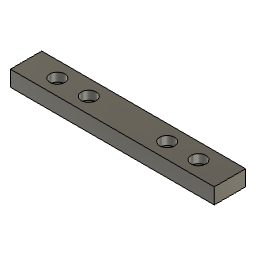
연습예제_1 (Autodesk Fusion 360 design; units mm, degrees)
Autodesk Fusion 360 part; units mm, degrees
sketch "Sketch1" plane through (0, 0, 0) normal (0, 0, 1) x (1, 0, 0)
  line L0 (-65, 20) -> (65, 20)
  line L1 (65, 20) -> (65, 0)
  line L2 (65, 0) -> (-65, 0)
  line L3 (-65, 0) -> (-65, 20)
  dimension "d1" = 130
  dimension "d2" = 20
  constraint horizontal L0
  constraint vertical L1
  constraint horizontal L2
  constraint vertical L3
  constraint midpoint origin L2
  measures "d1" distance of L0.start L0.end
  measures "d2" distance of L0.end L1.end
extrude "Extrude1" add sketch "Sketch1" along normal blind 10
sketch "Sketch3" plane through (0, 0, 10) normal (0, 0, 1) x (-1, 0, 0)
  line L0 (65, -20) -> (65, 0)
  line L1 (65, -10) -> (45, -10)
  line L2 (45, -10) -> (25, -10)
  line L3 (-65, 0) -> (-65, -20)
  line L4 (-65, -10) -> (-45, -10)
  line L5 (-45, -10) -> (-25, -10)
  point P0 (65, -20)
  dimension "d10" = 20
  dimension "d11" = 20
  dimension "d12" = 20
  dimension "d13" = 20
  constraint midpoint L0 L1.start
  constraint perpendicular L0 L1
  constraint parallel L1 L2
  constraint midpoint L3 L4.start
  constraint perpendicular L3 L4
  constraint parallel L4 L5
  measures "d10" distance of L1.start L1.end
  measures "d11" distance of L1.end L2.end
  measures "d12" distance of L4.start L4.end
  measures "d13" distance of L4.end L5.end
hole "Hole1" at (-45, 10, 10) at (25, 10, 10) at (45, 10, 10) at (-25, 10, 10) direction (0, 0, -1) diameter 5.029 depth 11 tip angle 118 counterbore diameter 9.5 counterbore depth 5.5
thread "Thread1" "ISO Metric profile 5.5 M5.5x0.5 6H" thread offset 0 thread depth 8.55
